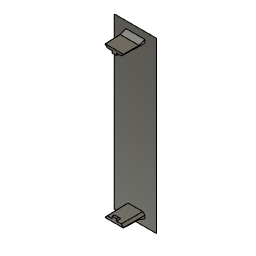
8080 End Caps (Autodesk Fusion 360 design; units mm, degrees)
Autodesk Fusion 360 part; units mm, degrees
sketch "Sketch1" plane through (0, 0, 0) normal (0, 1, 0) x (1, 0, 0)
  line L0 (10, 40) -> (-10, 40)
  line L1 (-10, 40) -> (-10, -40)
  line L2 (-10, -40) -> (10, -40)
  line L3 (10, -40) -> (10, 40)
  line L4 (10, 40) -> (-10, -40) construction
  line L5 (-10, 40) -> (10, -40) construction
  dimension "d1" = 20
  dimension "d2" = 80
  constraint horizontal L0
  constraint perpendicular L0 L1
  constraint parallel L0 L2
  constraint parallel L1 L3
  constraint coincident L4 origin
  constraint coincident L5 origin
  measures "d1" distance of L1.end L2.end
  measures "d2" distance of L0.end L1.end
extrude "Extrude1" add sketch "Sketch1" along normal blind 3
sketch "Sketch2" plane through (0, 0, 0) normal (0, -1, 0) x (1, 0, 0)
  line L0 (10, -40) -> (10, 40)
  line L1 (10, 40) -> (-10, 40)
  line L2 (-10, 40) -> (-10, -40)
  line L3 (-10, -40) -> (10, -40)
  line L4 (0, 48.0121) -> (0, -47.4969) construction
  line L5 (-22.9199, 34) -> (18.1137, 34) construction
  line L6 (-4.5, 35.75) -> (4.5, 35.75)
  line L7 (4.5, 35.75) -> (4.5, 34.25)
  line L8 (4.5, 34.25) -> (-4.5, 34.25)
  line L9 (-4.5, 34.25) -> (-4.5, 35.75)
  line L10 (29.4296, -34) -> (-24.7341, -34) construction
  line L11 (-4.5, -35.75) -> (4.5, -35.75)
  line L12 (4.5, -35.75) -> (4.5, -34.25)
  line L13 (4.5, -34.25) -> (-4.5, -34.25)
  line L14 (-4.5, -34.25) -> (-4.5, -35.75)
  dimension "d5" = 6
  dimension "d6" = 9
  dimension "d7" = 0.25
  dimension "d8" = 10
  dimension "d9" = 4.5
  dimension "d10" = 6
  dimension "d11" = 9
  dimension "d12" = 1.5
  dimension "d13" = 1.5
  dimension "d14" = 0.25
  dimension "d15" = 4.5
  constraint perpendicular L3 L4
  constraint perpendicular L0 L5
  constraint horizontal L6
  constraint vertical L7
  constraint horizontal L8
  constraint vertical L9
  constraint horizontal L10
  constraint horizontal L11
  constraint vertical L12
  constraint horizontal L13
  constraint vertical L14
  measures "d5" distance of L1 L5
  measures "d6" distance of L6.start L6.end
  measures "d7" distance of L5 L8
  measures "d8" distance of L2 L4
  measures "d9" distance of L4 L9
  measures "d10" distance of L3 L10
  measures "d11" distance of L11.start L11.end
  measures "d12" distance of L11.start L13.end
  measures "d13" distance of L6 L8
  measures "d14" distance of L10 L13
  measures "d15" distance of L4 L12
extrude "Extrude2" add sketch "Sketch2" along normal blind 10 draft -1 contours L6 L7 L8 L9 | L11 L12 L13 L14
chamfer "Chamfer1" distance 3 angle 45 4 edges at (-10, 3, 0) (0, 3, -40) (10, 3, 0) (0, 3, 40)
chamfer "Chamfer2" distance 1 angle 45 4 edges at (-4.4127, -5, -34.3373) (4.4127, -5, -34.3373) (-4.4127, -5, 34.3373) (4.4127, -5, 34.3373)
sketch "Sketch5" plane through (0, -10, 0) normal (0, -1, 0) x (1, 0, 0)
  line L0 (3.3253, 34.4246) -> (4.3254, 35.4247)
  line L1 (4.3254, 35.4247) -> (4.3254, 35.5754)
  line L2 (4.3254, 35.5754) -> (-4.3254, 35.5754)
  line L3 (-4.3254, 35.5754) -> (-4.3254, 35.4247)
  line L4 (-4.3254, 35.4247) -> (-3.3253, 34.4246)
  line L5 (-3.3253, 34.4246) -> (3.3253, 34.4246)
  line L6 (0, 34.4246) -> (1, 34.4246)
  line L7 (1, 34.4246) -> (1, 33.4246)
  line L8 (1, 33.4246) -> (0, 33.4246)
  line L9 (0, 33.4246) -> (0, 34.4246)
  line L10 (0, 34.4246) -> (-1, 34.4246)
  line L11 (-1, 34.4246) -> (-1, 33.4246)
  line L12 (-1, 33.4246) -> (0, 33.4246)
  line L13 (0, 33.4246) -> (0, 34.4246)
  dimension "d29" = 1
  dimension "d30" = 1
  dimension "d31" = 1
  constraint horizontal L6
  constraint vertical L7
  constraint horizontal L8
  constraint vertical L9
  constraint midpoint L5 L6.start
  constraint horizontal L10
  constraint vertical L11
  constraint horizontal L12
  constraint vertical L13
  measures "d29" distance of L6.start L6.end
  measures "d30" distance of L6.start L8.end
  measures "d31" distance of L6.start L8.end
sketch "Sketch6" plane through (0, -10, 0) normal (0, -1, 0) x (1, 0, 0)
  line L0 (4.3254, -35.4247) -> (3.3253, -34.4246)
  line L1 (3.3253, -34.4246) -> (-3.3253, -34.4246)
  line L2 (-3.3253, -34.4246) -> (-4.3254, -35.4247)
  line L3 (-4.3254, -35.4247) -> (-4.3254, -35.5754)
  line L4 (-4.3254, -35.5754) -> (4.3254, -35.5754)
  line L5 (4.3254, -35.5754) -> (4.3254, -35.4247)
  line L6 (0, -34.4246) -> (1, -34.4246)
  line L7 (1, -34.4246) -> (1, -33.4246)
  line L8 (1, -33.4246) -> (0, -33.4246)
  line L9 (0, -33.4246) -> (0, -34.4246)
  line L10 (0, -34.4246) -> (-1, -34.4246)
  line L11 (-1, -34.4246) -> (-1, -33.4246)
  line L12 (-1, -33.4246) -> (0, -33.4246)
  line L13 (0, -33.4246) -> (0, -34.4246)
  dimension "d32" = 1
  dimension "d33" = 1
  dimension "d34" = 1
  constraint horizontal L6
  constraint vertical L7
  constraint horizontal L8
  constraint vertical L9
  constraint midpoint L1 L6.start
  constraint horizontal L10
  constraint vertical L11
  constraint horizontal L12
  constraint vertical L13
  measures "d32" distance of L6.start L6.end
  measures "d33" distance of L6.start L8.end
  measures "d34" distance of L6.start L8.end
extrude "Extrude4" add sketch "Sketch5" sketch "Sketch6" against normal blind 2 contours L5 L6 L7 L8 L9 L13 | L5 L9 L10 L11 L12 L13 of sketch 2 contours L1 L6 L7 L8 L9 L13 | L1 L9 L10 L11 L12 L13
chamfer "Chamfer4" distance 0.9 angle 45 2 edges at (0, -8, -33.4246) (0, -8, 33.4246)
chamfer "Chamfer5" distance 1 angle 70 2 edges at (0, 0, 35.75) (0, 0, -35.75) measured on face at (1.1666, 0, 11.4167) measured on face at (1.1666, 0, 11.4167)
equation "d9 = d6 / 2"
equation "d15 = d11 / 2"
